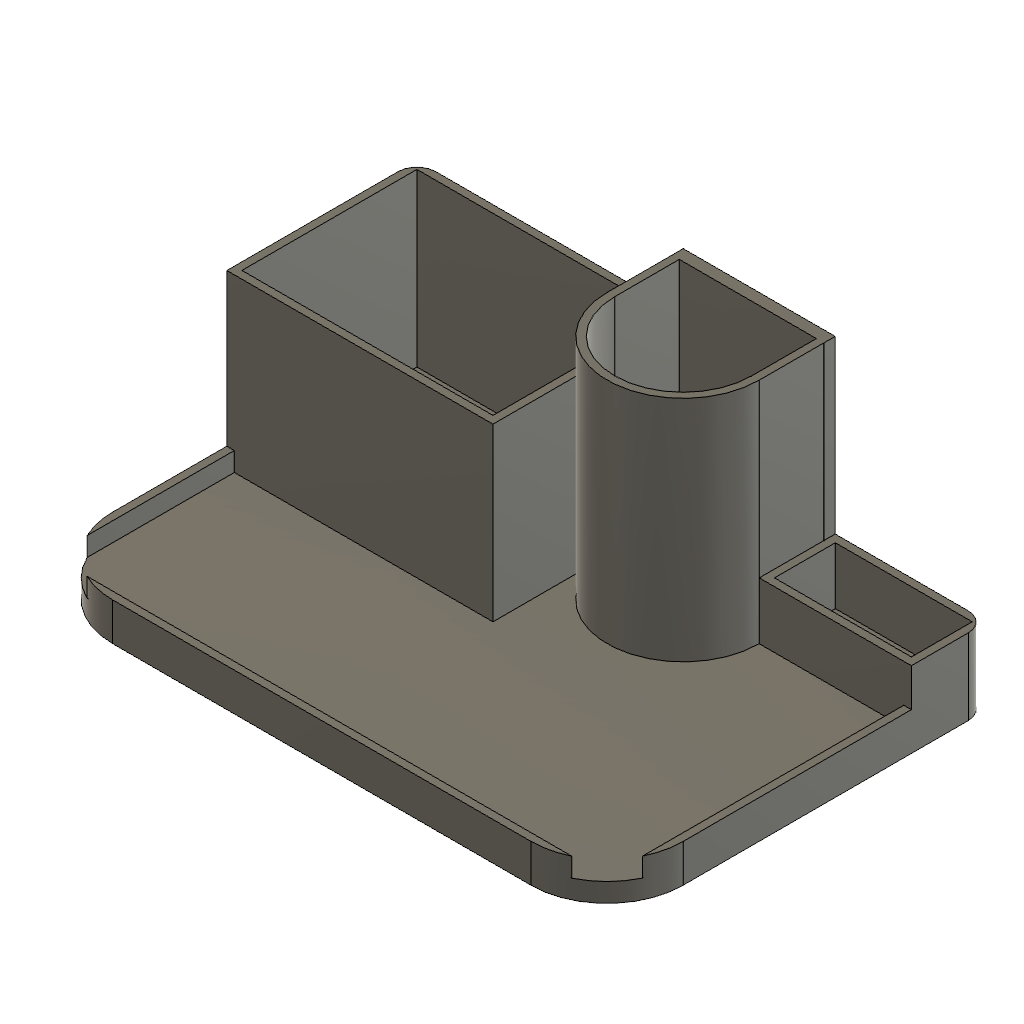
Desk Organiser (Autodesk Fusion 360 design; units mm, degrees)
part number: 2026-09-10-21-12-11-111
Autodesk Fusion 360 part; units mm, degrees
note: some values were not read from the file. Chosen so that the rebuilt part matches the saved one: which bodies a step acts on. Set by a fixed rule: which face or edge a step refers to.
sketch "Sketch1" plane through (0, 0, 0) normal (0, 1, 0) x (1, 0, 0)
  line L0 (-50, 50) -> (100, 50)
  line L1 (100, 50) -> (100, -50)
  line L2 (100, -50) -> (-50, -50)
  line L3 (-50, -50) -> (-50, 50)
  line L4 (-50, 0) -> (20, 0)
  line L5 (20, 0) -> (20, 50)
  line L6 (20, 50) -> (-50, 50)
  line L7 (-50, 50) -> (-50, 0)
  circle A0 centre (40, 30) radius 19.9828
  circle A1 centre (40, 30) radius 18.0191
  line L8 (60, 50) -> (100, 50)
  line L9 (100, 50) -> (100, 30)
  line L10 (100, 30) -> (60, 30)
  line L11 (60, 30) -> (60, 50)
  line L12 (62, 48) -> (98, 48)
  line L13 (98, 48) -> (98, 32)
  line L14 (98, 32) -> (62, 32)
  line L15 (62, 32) -> (62, 48)
  line L16 (18, 48) -> (-48, 48)
  line L17 (-48, 48) -> (-48, 2)
  line L18 (-48, 2) -> (18, 2)
  line L19 (18, 2) -> (18, 48)
  line L20 (-48, 0) -> (-48, -48)
  line L21 (-48, -48) -> (98, -48)
  line L22 (98, -48) -> (98, 30)
  constraint horizontal L0
  constraint vertical L1
  constraint horizontal L2
  constraint vertical L3
  constraint horizontal L4
  constraint vertical L5
  constraint horizontal L6
  constraint vertical L7
  constraint coincident L0 L5.end
  constraint midpoint L3 L4.start
  constraint concentric A0 A1
  constraint horizontal L8
  constraint vertical L9
  constraint horizontal L10
  constraint vertical L11
  constraint coincident L1 L9.end
  constraint coincident L0 L8.start
  constraint horizontal L12
  constraint vertical L13
  constraint horizontal L14
  constraint vertical L15
  constraint horizontal L16
  constraint vertical L17
  constraint horizontal L18
  constraint vertical L19
  constraint coincident L4 L20.start
  constraint perpendicular L4 L20
  constraint perpendicular L3 L21
  constraint coincident L10 L22.end
  constraint perpendicular L10 L22
extrude "Extrude1" add sketch "Sketch1" along normal blind 5 contours L0 L4 L5 L10 L11 L20 L21 L22 | A1 | L12 L13 L14 L15 | L16 L17 L18 L19 makes body 1 at (45.5398, 0, -30.8952) makes body 2 at (74, 0, -42.6667) makes body 3 at (-26, 0, -32.6667) makes body 4 at (23.3333, 0, 32)
extrude "Extrude2" add sketch "Sketch1" along normal blind 50 contours L0 L3 L4 L5 L6 L7 | A0 bodies 1 3 4
extrude "Extrude3" add sketch "Sketch1" along normal blind 20 contours L0 L1 L8 L9 L10 L11 bodies 1 2
extrude "Extrude4" add sketch "Sketch1" along normal blind 10 contours L1 L2 L3 L4 L10 L20 L21 L22 bodies 1
fillet "Fillet1" radius 20 2 edges at (100, 5, 50) (-50, 5, 50) on bodies 1
fillet "Fillet2" radius 5 1 edges at (-50, 25, -50) on bodies 1
fillet "Fillet3" radius 5 1 edges at (100, 10, -50) on bodies 1
sketch "Sketch2" plane through (0, 0, -50) normal (0, 0, -1) x (-1, 0, 0)
  line L0 (-95, 20) -> (-95, 0)
  line L1 (-95, 0) -> (45, 0)
  line L2 (45, 0) -> (45, 50)
  line L3 (45, 50) -> (-20, 50)
  line L4 (-20, 50) -> (-20, 5)
  line L5 (-20, 5) -> (-60, 5)
  line L6 (-60, 5) -> (-60, 20)
  line L7 (-60, 20) -> (-95, 20)
  line L8 (-20, 50) -> (-60, 50)
  line L9 (-60, 50) -> (-60, 3.0764)
  line L10 (-60, 3.0764) -> (-20, 3.0764)
  line L11 (-20, 3.0764) -> (-20, 50)
  constraint horizontal L8
  constraint vertical L9
  constraint horizontal L10
  constraint vertical L11
  constraint coincident L3.end L4.start
extrude "Extrude5" cut sketch "Sketch2" against normal blind 20 contours L4 L5 L6 L8 L9 L11 bodies 1
extrude "Extrude6" add 2 faces at (59.3282, 35, -30) (21.3263, 35, -30) along direction (0, 0, -1) blind 20 on bodies 1 bodies 1
extrude "Extrude7" add sketch "Sketch2" against normal blind 3 contours L4 L5 L6 L8 L9 L11 bodies 1
sketch "Sketch3" plane through (0, 50, 0) normal (0, 1, 0) x (-1, 0, 0)
  line L0 (-58.0191, -47) -> (-58.0191, -30)
  arc A0 (-21.9809, -30) -> (-58.0191, -30) centre (-40, -30) ccw
  line L1 (-21.9809, -30) -> (-21.9809, -47)
  line L2 (-21.9809, -47) -> (-58.0191, -47)
  arc A1 (45, -50) -> (50, -45) centre (45, -45) ccw
  line L3 (50, -45) -> (50, 0)
  line L4 (50, 0) -> (-20, 0)
  line L5 (-20, 0) -> (-20, -47)
  line L6 (-20, -47) -> (-20.0172, -47)
  line L7 (-20.0172, -47) -> (-20.0172, -30)
  arc A2 (-20.0172, -30) -> (-59.9828, -30) centre (-40, -30) ccw
  line L8 (-59.9828, -30) -> (-59.9828, -47)
  line L9 (-59.9828, -47) -> (-60, -47)
  line L10 (-60, -47) -> (-60, -50)
  line L11 (-60, -50) -> (45, -50)
  line L12 (-18, -48) -> (-18, -2)
  line L13 (-18, -2) -> (48, -2)
  line L14 (48, -2) -> (48, -48)
  line L15 (48, -48) -> (-18, -48)
  line L16 (-20.0172, -47) -> (-20, -50.5383)
  constraint coincident L6.end L7.start
extrude "Extrude8" add sketch "Sketch3" along normal blind 15 contours L7 A2 L8 L9 L10 L11 L16 bodies 1
